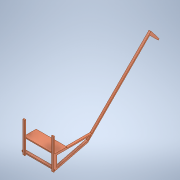
# Autodesk Inventor part: side1
Saved by Autodesk Inventor 2021.1 (Build 251245000, 245)
## iProperties
Created: 2020-09-07
Part Number: side1
Material: Wood (Walnut)
Document SubType Name: Modeling
Designer: robst
Density: 0.55 g/cm^3
Appearance: Walnut - Natural Polished
Author: robst
Autodesk Inventor part; units mm, degrees
ref_plane "YZ Plane" through (0, 0, 0) normal (1, 0, 0) x (0, 1, 0)
ref_plane "XZ Plane" through (0, 0, 0) normal (0, 1, 0) x (-1, 0, 0)
sketch "Sketch1" plane through (0, 0, 0) normal (1, 0, 0) x (0, 1, 0)
  line L0 (0, 0) -> (3228.5098, -3228.5098)
  line L1 (0, 0) -> (4565.8024, 0) construction
  line L2 (3228.5098, -3228.5098) -> (3192.5888, -3264.4309)
  line L3 (3192.5888, -3264.4309) -> (0, -71.842)
  line L4 (0, -71.842) -> (0, 0)
  line L5 (3192.5888, -3264.4309) -> (2708.0611, -3634.3566)
  line L6 (2708.0611, -3634.3566) -> (2677.2339, -3593.9793)
  line L7 (2677.2339, -3593.9793) -> (2671.5048, -3586.4752)
  line L8 (2671.5048, -3586.4752) -> (3093.0689, -3164.911)
  line L9 (0, 0) -> (-381, 1524)
  line L10 (-381, 1524) -> (-303.0467, 1543.4883)
  line L11 (-303.0467, 1543.4883) -> (110.4339, -110.4339)
  line L12 (0, 0) -> (23.9473, -95.7894)
  dimension "d0" = 4565.8024
  dimension "d1" = 45
  dimension "d2" = 50.8
  dimension "d3" = 609.6
  dimension "d4" = 50.8
  dimension "d5" = 381
  dimension "d6" = 1524
  constraints: 26 end point, 4 perpendicular, 4 point on line, 3 parallel, 1 equal length, 1 horizontal, 1 vertical
  measures "d0" distance of L0.start L0.end
  measures "d1" angle of L0 L1
  measures "d2" distance of L0.end L2.end
  measures "d3" distance of L2.end L5.end
  measures "d4" distance of L5.end L6.end
  measures "d5" horizontal distance of L9.end L0.start
  measures "d6" vertical distance of L9.end L0.start
extrude "Extrusion2" add sketch "Sketch1" along normal blind 101.6 contours L9 L10 L11 L0 | L0 L2 L3 L12 | L3 L5 L6 L7 L8
sketch "Sketch2" plane through (0, 0, 0) normal (-1, 0, 0) x (0, 0, 1)
  line L0 (1524, -381) -> (-95.7894, 23.9473) projected
  line L1 (1543.4883, -303.0467) -> (1524, -381) projected
  line L2 (-110.4339, 110.4339) -> (1543.4883, -303.0467) projected
  line L3 (1524, -381) -> (1425.4335, -356.3584)
  line L4 (1524, -381) -> (-95.7894, 23.9473) projected
  line L5 (1425.4335, -356.3584) -> (1444.9218, -278.4051)
  line L6 (-110.4339, 110.4339) -> (1543.4883, -303.0467) projected
  line L7 (1543.4883, -303.0467) -> (1524, -381) projected
  line L8 (1543.4883, -303.0467) -> (1524, -381)
  point P0 (0, 0)
  dimension "d11" = 101.6
  constraints: 6 end point, 2 point on line, 1 collinear, 1 perpendicular
  measures "d11" distance of L0.start L3.end
extrude "Extrusion3" add sketch "Sketch2" along normal blind 1524
sketch "Sketch3" plane through (101.6, 0, 0) normal (1, 0, 0) x (0, 0, -1)
  line L0 (110.4339, 110.4339) -> (-1543.4883, -303.0467) projected
  line L1 (-1543.4883, -303.0467) -> (-1543.4883, 306.5533)
  line L2 (-1543.4883, 306.5533) -> (-1441.8883, 306.5533)
  line L3 (-1441.8883, 306.5533) -> (-1441.8883, -277.6467)
  point P0 (0, 0)
  dimension "d14" = 609.6
  dimension "d15" = 101.6
  constraints: 6 end point, 1 horizontal, 1 perpendicular, 1 point on line, 1 vertical
  measures "d14" distance of L0.end L1.end
  measures "d15" distance of L1.end L2.end
extrude "Extrusion4" add sketch "Sketch3" against normal blind 101.6
sketch "Sketch4" plane through (101.6, -277.6467, 1441.8883) normal (0, 0, -1) x (-1, 0, 0)
  line L0 (0, 584.2) -> (101.6, 584.2) projected
  line L1 (101.6, -25.4) -> (101.6, 584.2) projected
  line L2 (0, 584.2) -> (101.6, 584.2)
  line L3 (101.6, 584.2) -> (101.6, 533.4)
  line L4 (101.6, 533.4) -> (0, 533.4)
  line L5 (0, 533.4) -> (0, 584.2)
  point P0 (101.6, 277.6467)
  dimension "d18" = 50.8
  constraints: 8 end point, 2 parallel, 1 horizontal, 1 perpendicular, 1 point on line
  measures "d18" distance of L2.end L3.end
extrude "Extrusion5" add sketch "Sketch4" along normal up to surface surface through (0, 3228.5098, -3228.5098) normal (0, 0.7071068, 0.7071068)
sketch "Sketch5" plane through (101.6, 0, 0) normal (1, 0, 0) x (0, 0, -1)
  line L0 (-1543.4883, 306.5533) -> (-933.8883, 306.5533)
  line L1 (-933.8883, 306.5533) -> (-933.8883, 357.3533)
  line L2 (-933.8883, 357.3533) -> (-1543.4883, 357.3533)
  line L3 (-1543.4883, 357.3533) -> (-1543.4883, 306.5533)
  point P0 (0, 0)
  dimension "d21" = 609.6
  dimension "d22" = 50.8
  constraints: 8 end point, 2 parallel, 1 horizontal, 1 perpendicular
  measures "d21" distance of L2.end L1.end
  measures "d22" distance of L1.end L0.end
extrude "Extrusion6" add sketch "Sketch5" against normal blind 1524
sketch "Sketch7" plane through (101.6, 357.3533, 1543.4883) normal (0, 1, 0) x (1, 0, 0)
  line L0 (0, 0) -> (-1524, 0) projected
  line L1 (-1524, 0) -> (-1524, 609.6) projected
  line L2 (-101.6, 0) -> (-1524, 0) projected
  line L3 (-1524, 0) -> (-1422.4, 0)
  line L4 (-1422.4, 0) -> (-1422.4, -50.8)
  line L5 (-1422.4, -50.8) -> (-1524, -50.8)
  line L6 (-1524, -50.8) -> (-1524, 0)
  point P0 (-101.6, 1543.4883)
  dimension "d25" = 101.6
  dimension "d26" = 50.8
  constraints: 8 end point, 2 parallel, 1 horizontal, 1 perpendicular
  measures "d25" distance of L4.end L5.end
  measures "d26" distance of L3.end L4.end
extrude "Extrusion7" add sketch "Sketch7" along normal mid plane 1524
ref_plane "Work Plane1" through (-660.4, 0, 0) normal (1, 0, 0) x (0, 0, -1)
mirror "Mirror1" about plane through (-660.4, 0, 0) normal (1, 0, 0) of "Extrusion7"
body "Solid2"
